Barrel - Printhead v1 (Autodesk Fusion 360 design; units mm, degrees)
Autodesk Fusion 360 part; units mm, degrees
sketch "Sketch1" plane through (0, 0, 0) normal (0, 1, 0) x (1, 0, 0)
  circle A0 centre (0, 0) radius 35
  dimension "d1" = 70
  constraint coincident A0.centre origin
  measures "d1" diameter of A0
extrude "Extrude1" add sketch "Sketch1" along normal blind 10 makes body 1
sketch "Sketch2" plane through (0, 10, 0) normal (0, 1, 0) x (-1, 0, 0)
  circle A0 centre (0, 0) radius 35
  circle A1 centre (0, 0) radius 20
  dimension "d4" = 40
  constraint coincident A0.centre A1.centre
  measures "d4" diameter of A1
extrude "Extrude2" add sketch "Sketch2" along normal blind 403 contours A1 bodies 1
sketch "Sketch3" plane through (0, 413, 0) normal (0, 1, 0) x (-1, 0, 0)
  circle A0 centre (0, 0) radius 20
sketch "Sketch4" plane through (0, 413, 0) normal (0, 1, 0) x (-1, 0, 0)
  circle A0 centre (0, 0) radius 12.5
  dimension "d7" = 25
  constraint coincident A0.centre origin
  measures "d7" diameter of A0
extrude "Extrude3" cut sketch "Sketch4" against normal blind 440 bodies 1
sketch "Sketch5" plane through (0, 0, 0) normal (0, -1, 0) x (1, 0, 0)
  circle A0 centre (0, 0) radius 12.5
  circle A1 centre (0, 0) radius 35
  circle A2 centre (0, 0) radius 20
  dimension "d10" = 40
  constraint coincident A0.centre A1.centre
  measures "d10" diameter of A2
extrude "Extrude4" add sketch "Sketch5" along normal blind 55 contours A2 bodies 1
sketch "Sketch6" plane through (0, 0, 0) normal (0, -1, 0) x (1, 0, 0)
  circle A0 centre (0, 0) radius 20
  circle A1 centre (0, 0) radius 35
  circle A2 centre (0, 27.5) radius 3
  circle A3 centre (-19.4454, 19.4454) radius 3
  circle A4 centre (-27.5, 0) radius 3
  circle A5 centre (-19.4454, -19.4454) radius 3
  circle A6 centre (0, -27.5) radius 3
  circle A7 centre (19.4454, -19.4454) radius 3
  circle A8 centre (27.5, 0) radius 3
  circle A9 centre (19.4454, 19.4454) radius 3
  dimension "d16" = 360
extrude "Extrude5" cut sketch "Sketch6" against normal blind 50 contours A2 | A3 | A4 | A5 | A6 | A7 | A8 | A9 bodies 1
sketch "Sketch7" plane through (0, 413, 0) normal (0, 1, 0) x (-1, 0, 0)
  circle A0 centre (0, 0) radius 12.5
  constraint coincident A0.centre origin
extrude "Extrude6" add sketch "Sketch7" against normal blind 468 separate body makes body 2
extrude "Extrude7" add 1 faces at (3.3879, -55, -0.621) along direction (0, -1, 0) blind 86 separate body on bodies 2 makes body 3
combine "Combine1" operation add target body 2 tool bodies 3
ref_plane "WorkPlane1" through (0, -81, 0) normal (0, -1, 0) x (1, 0, 0)
sketch "Sketch8" plane through (0, -81, 0) normal (0, -1, 0) x (1, 0, 0)
  circle A0 centre (0, 0) radius 9.925
  circle A1 centre (0, 0) radius 13
  dimension "d24" = 19.85
  dimension "d25" = 26
  constraint coincident A0.centre A1.centre
  measures "d24" diameter of A0
  measures "d25" diameter of A1
extrude "Extrude8" add sketch "Sketch8" along normal blind 10 separate body makes body 4
combine "Combine2" operation cut target body 2 tool bodies 4
equation "d16 = 360.0 °"
